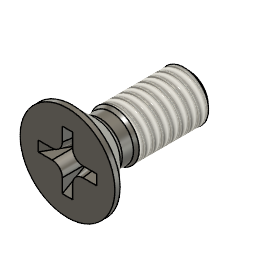
body (Autodesk Fusion 360 archive; units mm, degrees)
design "Countersunk Flat Head Screw ISO 7046-1 - M2.5 x 6 - H Steel 4.6 Plain"
description: Countersunk Flat Head Screw ISO 7046-1 - M2.5 x 6 - H
part number: ISO 7046-1 - M2.5 x 6 - H Steel 4.6 Plain
Autodesk Fusion 360 part; units mm, degrees
sketch "Sketch1" plane through (0, 0, 0) normal (0, 1, 0) x (1, 0, 0)
  line L0 (0, -2.612) -> (-2.35, -2.612)
  line L1 (-2.35, -2.612) -> (-2.35, -2.35)
  line L2 (-2.35, -2.35) -> (-1.112, -1.112)
  line L3 (-1.25, -0.212) -> (-1.25, 3.388)
  line L4 (-1.25, 3.388) -> (0, 3.388)
  line L5 (0, 3.388) -> (0, -2.612)
  line L6 (-1.112, -0.451) -> (-1.112, -1.112)
  line L7 (-1.25, -0.212) -> (-1.112, -0.451)
  dimension "d9" = 2.5
  dimension "d11" = 4.7
  dimension "d71" = 1.5
  dimension "d72" = 2.2239
  dimension "d89" = 3.6
  dimension "d101" = 30
  dimension "d115" = 6
  dimension "d121" = 45
  constraint perpendicular L0 L1
  constraint vertical L3
  constraint perpendicular L3 L4
  constraint perpendicular L0 L5
  constraint collinear origin L0.start L4.end
  constraint horizontal L0
  constraint coincident L2.end L6.end
  constraint coincident L6 L7.end
  constraint coincident L6.start L7.end
  constraint coincident origin L2
  measures "d71" distance of L0 L2.end
  measures "d89" distance of L4 L3.start
  measures "d101" angle of L3 L7
  measures "d115" distance of L0.start L4
  measures "d121" angle of L2 L5
revolve "Revolve1" add sketch "Sketch1" angle 360 about axis through (0, 0, -3.388) along (0, 0, 1) makes body 1
sketch "Sketch2" plane through (0, 0, 2.612) normal (0, 0, 1) x (1, 0, 0)
  line L0 (-0.255, 0.255) -> (-1.45, 0.255)
  line L1 (-1.45, 0.255) -> (-1.45, -0.255)
  line L2 (-1.45, -0.255) -> (-0.255, -0.255)
  line L3 (0.255, -1.45) -> (0.255, -0.255)
  line L4 (-0.255, -1.45) -> (0.255, -1.45)
  line L5 (-0.255, -0.255) -> (-0.255, -1.45)
  line L6 (1.45, 0.255) -> (0.255, 0.255)
  line L7 (1.45, -0.255) -> (1.45, 0.255)
  line L8 (0.255, -0.255) -> (1.45, -0.255)
  line L9 (-0.255, 1.45) -> (-0.255, 0.255)
  line L10 (0.255, 1.45) -> (-0.255, 1.45)
  line L11 (0.255, 0.255) -> (0.255, 1.45)
  dimension "d111" = 360
  dimension "d117" = 2.9
  dimension "d122" = 0.51
  constraint horizontal L0
  constraint perpendicular L0 L1
  constraint vertical L0.start L2.end
  constraint coincident L0.start L9.end
  measures "d117" distance of L4.start L10
  measures "d122" distance of L0 L2
extrude "Extrude1" add sketch "Sketch2" against normal blind 1.8 draft -4 separate body makes body 2
draft "Draft1" angle -30 neutral plane through (0, 0, 2.612) pull (0, 0, 1) 4 faces at (1.408, 0.043, 2.012) (-0.043, 1.408, 2.012) (-1.408, -0.043, 2.012) (-0.043, -1.408, 2.012) on bodies 2
fillet "Fillet3" radius 0.51 4 edges at (0.1921, 0.1921, 1.712) (0.1921, -0.1921, 1.712) (-0.1921, -0.1921, 1.712) (-0.1921, 0.1921, 1.712) on bodies 2
combine "Combine1" operation cut target body 1 tool bodies 2
thread "Thread1" "ISO Metric profile 2.5 M2.5x0.45 M2.5x0.45 6g" major diameter 2.43 minor diameter 1.9165 pitch 0.45 angle 60 resizes the face on face at (-1.2484, 0.0623, -0.988) on bodies 1
fillet "Fillet5" radius 0.25 1 edges at (-1.0367, 0.4021, 1.112) on bodies 1
sketch "Sketch6" plane through (0, 0, 0) normal (0, 1, 0) x (1, 0, 0)
  line L0 (-0.9739, 3.388) -> (-1.275, 3.388)
  line L1 (-1.275, 3.388) -> (-1.275, 3.112)
  line L2 (-1.275, 3.112) -> (-0.9739, 3.388)
  line L3 (-1.25, 3.388) -> (0, 3.388)
  line L4 (0, 0) -> (0, 3.388) construction
  dimension "d102" = 1.275
  dimension "d118" = 0.9739
  dimension "d119" = 0.2761
  constraint horizontal L0
  constraint perpendicular L0 L1
  constraint coincident L0.start L3
  constraint coincident L4.start origin
  constraint coincident L3.end L4.end
  measures "d102" distance of L4.start L1
  measures "d118" distance of L0.start L4
  measures "d119" distance of L0 L1.end
revolve "Revolve3" cut sketch "Sketch6" angle 360 about axis through (0, 0, 1.75) along (0, 0, 1) bodies 1
equation "d9 = adsk_nomdia"
equation "d11 = adsk_headdia"
equation "adsk_nomlen = 6.00 mm"
equation "adsk_headh = 1.50 mm"
equation "adsk_headdia = 4.70 mm"
equation "adsk_nomdia = 2.50 mm"
equation "adsk_headang = 90.00 deg"
equation "adsk_phildia = 2.90 mm"
equation "d31 = -adsk_phildepth"
equation "adsk_philwidth = 0.51 mm"
equation "adsk_phildepth = 1.80 mm"
equation "d71 = adsk_headh"
equation "d72 = adsk_shnkdia"
equation "adsk_shnkdia = 2.2239475 mm"
equation "d89 = adsk_thrlen"
equation "adsk_thrlen = 3.60 mm"
equation "adsk_pitch1 = 0.45 mm"
equation "adsk_startlen = 0.2760525 mm"
equation "adsk_midfillet = adsk_nomdia * 0.1"
equation "d96 = adsk_midfillet"
equation "d99 = ( adsk_shnkdia / 2 ) * tan(90 deg - adsk_headang / 2) + adsk_headh"
equation "d102 = adsk_nomdia * 0.51"
equation "adsk_endpointdia = 1.947895 mm"
equation "d114 = adsk_philwidth"
equation "d115 = adsk_nomlen"
equation "d117 = adsk_phildia"
equation "d118 = adsk_endpointdia / 2"
equation "d119 = adsk_startlen"
equation "d121 = adsk_headang * 0.5"
equation "d122 = adsk_philwidth"
